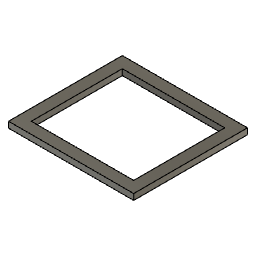
spacer+2mm (Autodesk Fusion 360 design; units mm, degrees)
Autodesk Fusion 360 part; units mm, degrees
sketch "Sketch1" plane through (0, 0, 0) normal (0, 0, 1) x (1, 0, 0)
  line L0 (0, 0) -> (41.91, 0)
  line L1 (41.91, 0) -> (41.91, 38.1)
  line L2 (41.91, 38.1) -> (0, 38.1)
  line L3 (0, 38.1) -> (0, 0)
  line L4 (0, 38.1) -> (3.81, 38.1)
  line L5 (3.81, 34.29) -> (3.81, 3.81)
  line L6 (0, 0) -> (0, 3.81)
  line L7 (3.81, 3.81) -> (38.1, 3.81)
  line L8 (0, 38.1) -> (0, 34.29)
  line L9 (3.81, 34.29) -> (38.1, 34.29)
  line L10 (41.91, 38.1) -> (38.1, 38.1)
  line L11 (38.1, 34.29) -> (38.1, 3.81)
  dimension "d1" = 41.91
  dimension "d2" = 38.1
  dimension "d3" = 3.81
  dimension "d4" = 3.81
  dimension "d5" = 3.81
  dimension "d6" = 3.81
  constraint horizontal L0
  constraint vertical L1
  constraint horizontal L2
  constraint vertical L3
  constraint coincident L0.start L3.end
  constraint perpendicular L3 L4
  constraint perpendicular L0 L5
  constraint perpendicular L0 L6
  constraint perpendicular L1 L7
  constraint perpendicular L4 L8
  constraint perpendicular L1 L9
  constraint perpendicular L1 L10
  constraint perpendicular L0 L11
  measures "d1" distance of L0.start L0.end
  measures "d2" distance of L0.start L2.end
  measures "d3" distance of L2.end L4.end
  measures "d4" distance of L0.start L6.end
  measures "d5" distance of L2.end L8.end
  measures "d6" distance of L1.end L10.end
sketch "Sketch2" plane through (0, 0, 0) normal (0, 0, 1) x (1, 0, 0)
extrude "Extrude1" add sketch "Sketch1" along normal blind 2
